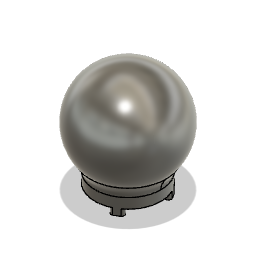
Modified Bulb Lamp v3 (Autodesk Fusion 360 design; units mm, degrees)
Autodesk Fusion 360 part; units mm, degrees
sketch "Sketch1" plane through (0, 0, 0) normal (0, 0, 1) x (1, 0, 0)
  circle A0 centre (-15.218416, 19.599615) radius 19.6
  line L0 (-15.35, 39.199174) -> (-15.35, 42.09923)
  line L1 (-15.35, -2.9) -> (-15.35, 42.09923) construction
  line L2 (-2.6, 0) -> (-2.6, 4.601763)
  line L3 (-2.6, -7.675) -> (-2.6, 0)
  line L4 (-2.6, 0) -> (-4.168299, 0)
  line L5 (0, 0) -> (-15.35, 0)
  line L6 (0, 0) -> (-2.6, 0) construction
  line L7 (0, 0) -> (0, -7.675)
  line L8 (-15.35, 0) -> (-15.35, -2.9)
  line L9 (0, -7.675) -> (-2.6, -7.675)
  spline S0 degree 2 poles (0, 0) (0, 1.865078) (2.152823, 5.299613) knots 0 0 0 0.58045235 0.58045235 0.58045235 weights 1 2.09889315 1
  arc A1 (2.152823, 5.299613) -> (-2.6, 0.970993) centre (-15.218416, 19.599615) ccw
  dimension "d1" = 2.9
  dimension "d2" = 45
  dimension "d3" = 7.675
  dimension "d4" = 2.6
  dimension "d5" = 39.2
  dimension "d6" = 15.35
  constraint coincident L5.start L6.start
  constraint coincident L5.end L8.start
  constraint coincident L1.start A1
  constraint perpendicular L1 L5
  constraint vertical L7
  constraint perpendicular L1 L9
  constraint coincident L2.start L5
  constraint perpendicular L6 L7
  constraint perpendicular L3 L5
  constraint collinear L1 L8
  constraint concentric A0 A1
  constraint perpendicular L2 L6
  measures "d1" distance of L5.end L1.start
  measures "d2" diameter of A1
  measures "d3" distance of L5.start L7.end
  measures "d4" horizontal distance of L3.start L7.end
  measures "d5" diameter of A0
  measures "d6" horizontal distance of L5.end L5.start
revolve "Revolve1" add sketch "Sketch1" angle 360 about axis through (-15.35, -2.9, 0) along (0, 1, 0) contours A0 L0 L2 L5 S0 A1 | L3 L5 L7 L9 picked at (-1.617549, 2.563687) picked at (-1.733333, -2.558333)
sketch "Sketch2" plane through (0, -7.675, 0) normal (0, -1, 0) x (1, 0, 0)
  circle A0 centre (-15.35, 0) radius 15.35
  circle A1 centre (-15.35, 0) radius 12.75
  line L0 (-15.35, 0) -> (-15.081416, 15.34765)
  line L1 (-15.35, 0) -> (-26.01251, 11.042345)
  line L2 (-15.35, 0) -> (-30.69765, 0.268584)
  line L3 (-15.35, 0) -> (-26.392345, -10.66251)
  line L4 (-15.35, 0) -> (-15.618584, -15.34765)
  line L5 (-15.35, 0) -> (-4.68749, -11.042345)
  line L6 (-15.35, 0) -> (-0.00235, -0.268584)
  line L7 (-15.35, 0) -> (-4.307655, 10.66251)
  circle A2 centre (-15.35, 0) radius 12.75
  circle A3 centre (-15.35, 0) radius 15.35
  line L8 (-6.9009, 9.548571) -> (-5.002281, 11.381881) construction
  arc A4 (-8.629956, 13.800852) -> (-9.768205, 11.463248) centre (-9.199081, 12.63205) ccw
  arc A5 (-7.751566, 10.238471) -> (-6.202081, 12.326316) centre (-6.976823, 11.282394) ccw
  dimension "d11" = 2.6
  dimension "d12" = 2.6
  dimension "d13" = 45
  constraint coincident A0.centre A1.centre
  constraint concentric A2 A3
  constraint tangent A0 A3
  constraint tangent A1 A2
  constraint tangent A2 A5
  constraint tangent L8 A5
  constraint tangent A4 A5
  constraint tangent A3 A4
  measures "d11" diameter of A5
  measures "d12" diameter of A4
  measures "d13" angle of L0 L8
extrude "Extrude1" cut sketch "Sketch2" against normal blind 3 contours A0 A1 L7 A2 A3 A5 | A0 A1 L0 A2 A3 A4 | A0 A1 L0 L1 A2 A3 picked at (-5.49313, 9.983599) picked at (-12.281892, 14.118953) picked at (-24.475339, 11.210491)
pattern_circular "C-Pattern1" count 4 over 360 about axis through (-15.35, 19.599615, 0) along (0, -1, 0) of "Extrude1"
equation "d1 = Thickness_Joint"
equation "d3 = d899 / 2"
